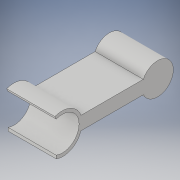
# Autodesk Inventor part: turtlearm
Saved by Autodesk Inventor 2018 (Build 220112000, 112)
## iProperties
Created: 2017-10-25
Part Number: turtlearm
Material: Generic
Document SubType Name: Modeling
Designer: kcmat
Density: 1 g/cm^3
Appearance: Default
Author: kcmat
Autodesk Inventor part; units mm, degrees
ref_plane "YZ Plane" through (0, 0, 0) normal (1, 0, 0) x (0, 1, 0)
ref_plane "XZ Plane" through (0, 0, 0) normal (0, 1, 0) x (-1, 0, 0)
ref_plane "XY Plane" through (0, 0, 0) normal (0, 0, 1) x (1, 0, 0)
sketch "Sketch1" plane through (0, 0, 0) normal (1, 0, 0) x (0, 1, 0)
  arc A0 (-3.0896, 1.1338) -> (3.0896, 1.1338) centre (0, -0.0687) ccw
  line L0 (-3.0896, 1.1338) -> (-3.3549, 1.1338)
  line L1 (3.0896, 1.1338) -> (3.3102, 1.2365)
  circle A1 centre (-0.026, -18.9035) radius 3.1136
  arc A2 (1.2951, -16.0841) -> (-1.3472, -16.0841) centre (-0.026, -18.9035) ccw
  line L2 (3.0896, 1.1338) -> (3.6653, 1.4017)
  line L3 (-3.0896, 1.1338) -> (-3.7246, 1.1338)
  arc A3 (-3.7246, 1.1338) -> (-1.3472, -3.7376) centre (-0.2877, -0.2047) ccw
  arc A4 (1.2951, -3.7556) -> (3.6653, 1.4017) centre (-0.0687, -0.0056) ccw
  line L4 (1.2951, -3.7556) -> (1.2951, -16.0841)
  line L5 (-1.3472, -16.0841) -> (-1.3472, -3.7376)
  point P0 (0, 0)
  dimension "d12" = 0.635
  dimension "d13" = 0.635
  constraints: 12 end point, 8 point on circle, 4 centre point, 2 horizontal, 1 parallel, 4 other
  measures "d12" distance of L1.start L2.end
  measures "d13" distance of L0.start L3.end
extrude "Extrusion3" add sketch "Sketch1" along normal blind 9.525
body "Solid3"
